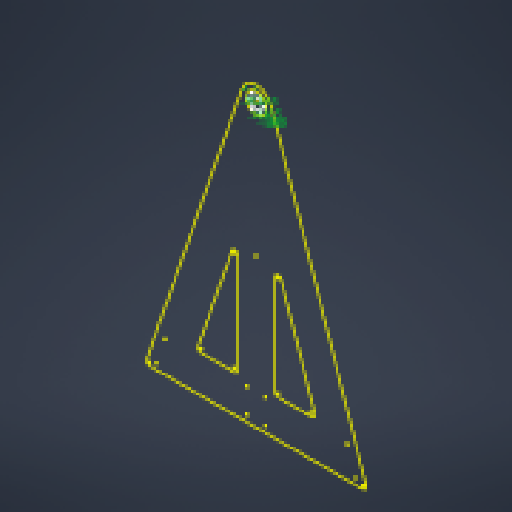
# Autodesk Inventor part: MainOuterBearingMount
Saved by Autodesk Inventor 2024.1 (Build 281209000, 209)
## iProperties
Created: 2023-10-16
Part Number: MainOuterBearingMount
Material: Generic
Document SubType Name: Modeling
Designer: Brandon
Density: 1 g/cm^3
Appearance: Default
Author: Brandon
Autodesk Inventor part; units mm, degrees
ref_plane "YZ Plane" through (0, 0, 0) normal (1, 0, 0) x (0, 1, 0)
ref_plane "XZ Plane" through (0, 0, 0) normal (0, 1, 0) x (-1, 0, 0)
ref_plane "XY Plane" through (0, 0, 0) normal (0, 0, 1) x (1, 0, 0)
sketch "Sketch1" plane through (0, 0, 0) normal (0, 0, 1) x (1, 0, 0)
  circle A0 centre (0, 273.05) radius 20.955 projected
  circle A1 centre (0, 273.05) radius 11 projected
  arc A2 (219.754, -304.8) -> (225.7704, -296.4188) centre (219.754, -298.45) ccw projected
  line L0 (225.7704, -296.4188) -> (30.0819, 283.206) projected
  arc A3 (30.0819, 283.206) -> (-30.0819, 283.206) centre (0, 273.05) ccw projected
  line L1 (-30.0819, 283.206) -> (-225.7704, -296.4188) projected
  arc A4 (-225.7704, -296.4188) -> (-219.754, -304.8) centre (-219.754, -298.45) ccw projected
  line L2 (-219.754, -304.8) -> (219.754, -304.8) projected
  line L3 (-38.1, -17.4222) -> (-38.1, -222.25) projected
  arc A5 (-44.45, -228.6) -> (-38.1, -222.25) centre (-44.45, -222.25) ccw projected
  line L4 (-44.45, -228.6) -> (-113.6024, -228.6) projected
  arc A6 (-119.6188, -220.2188) -> (-113.6024, -228.6) centre (-113.6024, -222.25) ccw projected
  line L5 (-119.6188, -220.2188) -> (-50.4664, -15.391) projected
  arc A7 (-38.1, -17.4222) -> (-50.4664, -15.391) centre (-44.45, -17.4222) ccw projected
  line L6 (113.6024, -228.6) -> (44.45, -228.6) projected
  arc A8 (38.1, -222.25) -> (44.45, -228.6) centre (44.45, -222.25) ccw projected
  line L7 (38.1, -222.25) -> (38.1, -17.4222) projected
  arc A9 (50.4664, -15.391) -> (38.1, -17.4222) centre (44.45, -17.4222) ccw projected
  line L8 (50.4664, -15.391) -> (119.6188, -220.2188) projected
  arc A10 (113.6024, -228.6) -> (119.6188, -220.2188) centre (113.6024, -222.25) ccw projected
  circle A11 centre (-204.2059, -292.1) radius 2 projected
  circle A12 centre (-187.0552, -241.3) radius 2 projected
  circle A13 centre (187.0552, -241.3) radius 2 projected
  circle A14 centre (204.2059, -292.1) radius 2 projected
  circle A15 centre (19.05, -241.3) radius 2 projected
  circle A16 centre (19.05, -292.1) radius 2 projected
  circle A17 centre (-19.05, -292.1) radius 2 projected
  circle A18 centre (-19.05, -241.3) radius 2 projected
  circle A19 centre (8.255, 287.3481) radius 2 projected
  circle A20 centre (-8.255, 287.3481) radius 2 projected
  circle A21 centre (-16.51, 273.05) radius 2 projected
  circle A22 centre (-8.255, 258.7519) radius 2 projected
  circle A23 centre (8.255, 258.7519) radius 2 projected
  circle A24 centre (16.51, 273.05) radius 2 projected
  circle A25 centre (0, 273.05) radius 11 projected
  circle A26 centre (0, 273.05) radius 11.0762
  circle A27 centre (-8.255, 287.3481) radius 2.1
  circle A28 centre (8.255, 287.3481) radius 2.1
  circle A29 centre (16.51, 273.05) radius 2.1
  circle A30 centre (8.255, 258.7519) radius 2.1
  circle A31 centre (-8.255, 258.7519) radius 2.1
  circle A32 centre (-16.51, 273.05) radius 2.1
  circle A33 centre (0, 273.05) radius 4.35
  point P0 (0, 0)
  dimension "d0" = 0.0762
  dimension "d1" = 4.2
  dimension "d2" = 4.2
  dimension "d3" = 4.2
  dimension "d4" = 4.2
  dimension "d5" = 4.2
  dimension "d6" = 4.2
  dimension "d9" = 8.7
  constraints: 8 centre point, 7 coincident
  measures "d0" radial gap between concentric circles of A1 A26
  measures "d1" diameter of A27
  measures "d2" diameter of A28
  measures "d3" diameter of A29
  measures "d4" diameter of A30
  measures "d5" diameter of A31
  measures "d6" diameter of A32
  measures "d9" diameter of A33
extrude "Extrusion1" add sketch "Sketch1" along normal blind 7.015 contours A0 | A1 | A26
extrude "Extrusion2" cut sketch "Sketch1" along normal blind 4.475 contours A1 | A26 | A33
chamfer "Chamfer1" distance 0.635 angle 45 7 edges at (-11.0762, 273.05, 4.475) (6.155, 287.3481, 7.015) (-10.355, 287.3481, 7.015) (-18.61, 273.05, 7.015) (-10.355, 258.7519, 7.015) (6.155, 258.7519, 7.015) (14.41, 273.05, 7.015)
body "Solid1"
